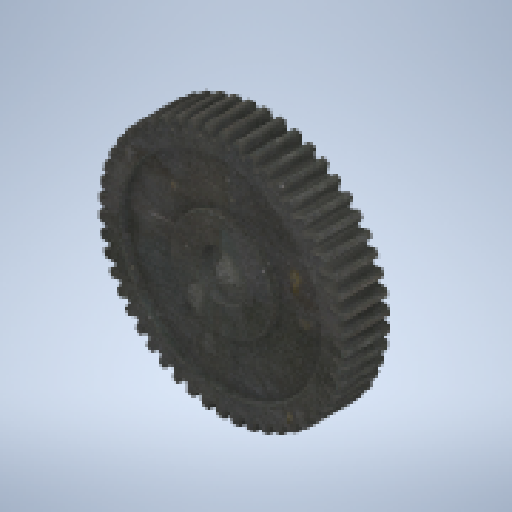
# Autodesk Inventor part: Engranaje recto2
Saved by Autodesk Inventor 2024 (Build 280153000, 153)
## iProperties
CustomPartVersion: 0
Created: 2023-12-10
Part Number: Engranaje recto2
Material: Acero
Document SubType Name: Modeling
Designer: Jhon
Categories: <?xml version="1.0" encoding="UTF-16"?> <MemberInstance><Categories><FamilyTemplate><FamilyTemplateParameter ValueType="xs:double" Id="1" ObjectReferenceKey="da_z" ObjectType="kUserParameterObject"/><FamilyTemplateParameter ValueType="xs:double" Id="2" ObjectReferenceKey="da_b" ObjectType="kUserParameterObject"/><FamilyTemplateParameter ValueType="xs:double" Id="3" ObjectReferenceKey="da_beta" ObjectType="kUserParameterObject"/><FamilyTemplateParameter ValueType="xs:double" Id="4" ObjectReferenceKey="da_da" ObjectType="kUserParameterObject"/><FamilyTemplateParameter ValueType="xs:double" Id="5" ObjectReferenceKey="da_aw" ObjectType="kUserParameterObject"/><FamilyTemplateParameter ValueType="xs:string" Id="6" ObjectReferenceKey="EAIAABAAAACIAQAAAAAAAIAAAAAAAAAA" ObjectType="83910656" SubObjectId="SurfaceGeometry"/></FamilyTemplate><ParamToTemplateMap><ParamToTemplate CategoryParameter="//CategoryParameter[@InternalName='046C89C9-8512-4d59-83FE-43B91F4F132A']" TemplateParameter="1"/><ParamToTemplate CategoryParameter="//CategoryParameter[@InternalName='2552DF32-E462-4b46-AEBF-C6C7768E72AC']" TemplateParameter="2"/><ParamToTemplate CategoryParameter="//CategoryParameter[@InternalName='C9EE641D-15FC-4fae-A226-E94C4372FDD7']" TemplateParameter="3"/><ParamToTemplate><ParamToTemplate CategoryParameter="//CategoryParameter[@InternalName='00B6519A-459B-49c7-AD84-2E56D39A5744']" ConstantValue="0.000000"/></ParamToTemplate><ParamToTemplate><ParamToTemplate CategoryParameter="//CategoryParameter[@InternalName='04B31F0E-C7A6-4894-AA32-9629BEFACF47']" ConstantValue="1.000000"/></ParamToTemplate><ParamToTemplate><ParamToTemplate CategoryParameter="//CategoryParameter[@InternalName='43CBEC2E-7847-49e7-A936-2F7889FCB2D9']" ConstantValue="0.250000"/></ParamToTemplate><ParamToTemplate><ParamToTemplate CategoryParameter="//CategoryParameter[@InternalName='B1EFC894-105D-4ebd-86BF-FA20ED196853']" ConstantValue="0.337200"/></ParamToTemplate><ParamToTemplate><ParamToTemplate CategoryParameter="//CategoryParameter[@InternalName='51175063-3D10-4879-93E8-6246FE8B403D']" ConstantValue="2060000000.000000"/></ParamToTemplate><ParamToTemplate><ParamToTemplate CategoryParameter="//CategoryParameter[@InternalName='A3A52E27-4454-46a9-B0BD-C932399B70AF']" ConstantValue="0.300000"/></ParamToTemplate><ParamToTemplate><ParamToTemplate CategoryParameter="//CategoryParameter[@InternalName='91B76062-C214-41d9-B1B9-14D2AB99603D']" ConstantValue="0.400000"/></ParamToTemplate><ParamToTemplate><ParamToTemplate CategoryParameter="//CategoryParameter[@InternalName='374E806E-8B8A-4dda-A9AA-1039D6500AD2']" ConstantValue="2.500000"/></ParamToTemplate><ParamToTemplate><ParamToTemplate CategoryParameter="//CategoryParameter[@InternalName='2D373A89-B862-43d6-8D0B-0CBF12AB9F6C']" ConstantValue="0.349066"/></ParamToTemplate><ParamToTemplate CategoryParameter="//CategoryParameter[@InternalName='37777632-D6A2-4fac-9D53-DB8ACD95C989']" TemplateParameter="4"/><ParamToTemplate CategoryParameter="//CategoryParameter[@InternalName='FD1017F1-B727-4f7e-9707-0F86F1FF9423']" TemplateParameter="5"/><ParamToTemplate><ParamToTemplate CategoryParameter="//CategoryParameter[@InternalName='9E1B4470-B2D3-4ff1-B813-535BB4CDF51A']" ConstantValue="3520000.000000"/></ParamToTemplate><ParamToTemplate><ParamToTemplate CategoryParameter="//CategoryParameter[@InternalName='F8452263-BFF6-458c-9FB1-07C4B99E95CD']" ConstantValue="11400000.000000"/></ParamToTemplate><ParamToTemplate><ParamToTemplate CategoryParameter="//CategoryParameter[@InternalName='3E3BB259-FD49-497f-8171-6EBC954A3479']" ConstantValue="2.000000"/></ParamToTemplate><ParamToTemplate CategoryParameter="//CategoryParameter[@InternalName='27C3BAF2-7550-4e4b-AE2C-0DB134B7D9B7']" TemplateParameter="6"/></ParamToTemplateMap><Category DisplayName="Gear" InternalName="DC85795E-93AB-48d5-8EEE-5A27447B64BD" Mnemonic="Gear"><CategoryParameter DisplayName="z" InternalName="046C89C9-8512-4d59-83FE-43B91F4F132A" Mnemonic="z"/><CategoryParameter DisplayName="b" InternalName="2552DF32-E462-4b46-AEBF-C6C7768E72AC" Mnemonic="b"/><CategoryParameter DisplayName="||b|" InternalName="C9EE641D-15FC-4fae-A226-E94C4372FDD7" Mnemonic="beta"/><CategoryParameter DisplayName="x" InternalName="00B6519A-459B-49c7-AD84-2E56D39A5744" Mnemonic="x"/><CategoryParameter DisplayName="a*" InternalName="04B31F0E-C7A6-4894-AA32-9629BEFACF47" Mnemonic="a"/><CategoryParameter DisplayName="c*" InternalName="43CBEC2E-7847-49e7-A936-2F7889FCB2D9" Mnemonic="c"/><CategoryParameter DisplayName="r|.f|*" InternalName="B1EFC894-105D-4ebd-86BF-FA20ED196853" Mnemonic="rf"/><CategoryParameter DisplayName="E" InternalName="51175063-3D10-4879-93E8-6246FE8B403D" Mnemonic="E"/><CategoryParameter DisplayName="||m|" InternalName="A3A52E27-4454-46a9-B0BD-C932399B70AF" Mnemonic="mi"/><Category DisplayName="SpurGear" InternalName="26C5A22E-A91E-4dfd-A3B3-23CCAFAE1764" Mnemonic="SpurGear"><CategoryParameter DisplayName="m" InternalName="91B76062-C214-41d9-B1B9-14D2AB99603D" Mnemonic="m"/><CategoryParameter DisplayName="P" InternalName="374E806E-8B8A-4dda-A9AA-1039D6500AD2" Mnemonic="PP"/><CategoryParameter DisplayName="||a|" InternalName="2D373A89-B862-43d6-8D0B-0CBF12AB9F6C" Mnemonic="alpha"/><CategoryParameter DisplayName="d|.a|" InternalName="37777632-D6A2-4fac-9D53-DB8ACD95C989" Mnemonic="da"/><CategoryParameter DisplayName="a|.w|" InternalName="FD1017F1-B727-4f7e-9707-0F86F1FF9423" Mnemonic="aw"/><CategoryParameter DisplayName="||s||.Flim|" InternalName="9E1B4470-B2D3-4ff1-B813-535BB4CDF51A" Mnemonic="sFlim"/><CategoryParameter DisplayName="||s||.Hlim|" InternalName="F8452263-BFF6-458c-9FB1-07C4B99E95CD" Mnemonic="sHlim"/><CategoryParameter DisplayName="tipo" InternalName="3E3BB259-FD49-497f-8171-6EBC954A3479" Mnemonic="type"/><CategoryParameter DisplayName="PitchDiameter" InternalName="27C3BAF2-7550-4e4b-AE2C-0DB134B7D9B7" Mnemonic="IDS_PITCHDIAM"/></Category></Category></Categories></MemberInstance>
Mass: 8265.26 g
Surface Area: 1323.38 cm^2
Volume: 1052.9 cm^3
Density: 7.85 g/cm^3
Appearance: Placa
Author: Jhon
Autodesk Inventor part; units mm, degrees
sketch "Sketch1" plane through (0, 0, 0) normal (0, 0, 1) x (1, 0, 0)
  circle A0 centre (0, 0) radius 104
  dimension "d0" = 208
  constraints: 1 centre point
  measures "d0" diameter of A0
extrude "Extrusion1" add sketch "Sketch1" along normal blind 40
ref_plane "Work Plane2" through (0, 0, 20) normal (0, 0, 1) x (1, 0, 0)
sketch "Sketch2" plane through (0, 0, 0) normal (0, 0, -1) x (-1, 0, 0)
  circle A0 centre (0, 0) radius 104 projected
  circle A1 centre (0, 0) radius 100
  dimension "d3" = 200
  constraints: 1 centre point, 1 coincident
  measures "d3" diameter of A1
surface extrude "Diámetro de separación" sketch "Sketch2" against normal through all shown no curves A1
ref_plane "Work Plane8" through (0, 0, 0) normal (0.9980267, 0.0627905, 0) x (0, 0, 1)
ref_plane "Work Plane9" through (0, 0, 0) normal (1, 0, 0) x (0, 1, 0)
spur gear teeth "Engranaje recto" teeth 50 pitch diameter 200 tip diameter 208 root diameter 190 face width 40 start plane through (0, 0, 0) normal (0, 0, -1) x (-1, 0, 0)
sketch "Boceto3" plane through (0, 0, 0) normal (0, 0, -1) x (-1, 0, 0)
  arc A0 (-18.0702, -8.5714) -> (-18.0702, 8.5714) centre (0, 0) ccw
  circle A1 centre (0, 0) radius 42.5
  circle A2 centre (0, 0) radius 84
  line L0 (-22.721, -8.5714) -> (-18.0702, -8.5714)
  line L1 (-18.0702, 8.5714) -> (-22.721, 8.5714)
  line L2 (-22.721, 8.5714) -> (-22.721, -8.5714)
  dimension "d49" = 40
  dimension "d50" = 85
  dimension "d53" = 168
  constraints: 6 end point, 3 centre point, 3 coincident, 2 point on circle, 1 horizontal, 1 parallel
  measures "d49" diameter of A0
  measures "d50" diameter of A1
  measures "d53" diameter of A2
sketch "Boceto5" plane through (0, 0, 40) normal (0, 0, 1) x (1, 0, 0)
  circle A0 centre (0, 0) radius 84
  circle A1 centre (0, 0) radius 42.5
  dimension "d67" = 168
  dimension "d68" = 85
  constraints: 2 centre point, 2 coincident
  measures "d67" diameter of A0
  measures "d68" diameter of A1
extrude "Extrusión6" add sketch "Boceto3" along normal blind 20 contours A1
extrude "Extrusión7" cut sketch "Boceto3" against normal blind 40 contours L0 L2 L1 A0
extrude "Extrusión8" cut sketch "Boceto3" against normal blind 7 contours A2
extrude "Extrusión9" cut sketch "Boceto5" against normal blind 7
chamfer "Chaflán2" distance 2 angle 45 50 edges at (103.7948, 6.5302, 0) (103.7948, -6.5302, 0) (102.1579, 19.4877, 0) (102.1579, -19.4877, 0) (98.9099, 32.1378, 0) (98.9099, -32.1378, 0) (94.102, 44.281, 0) (94.102, -44.281, 0) (87.8101, 55.726, 0) (87.8101, -55.726, 0) (80.1334, 66.2921, 0) (80.1334, -66.2921, 0) (71.1929, 75.8127, 0) (71.1929, -75.8127, 0) (61.1297, 84.1378, 0) (61.1297, -84.1378, 0) (50.1024, 91.1359, 0) (50.1024, -91.1359, 0) (38.285, 96.6968, 0) (38.285, -96.6968, 0) (25.8637, 100.7326, 0) (25.8637, -100.7326, 0) (13.0347, 103.1799, 0) (13.0347, -103.1799, 0) (0, 104, 0) (0, -104, 0) (-13.0347, 103.1799, 0) (-13.0347, -103.1799, 0) (-25.8637, 100.7326, 0) (-25.8637, -100.7326, 0) (-38.285, 96.6968, 0) (-38.285, -96.6968, 0) (-50.1024, 91.1359, 0) (-50.1024, -91.1359, 0) (-61.1297, 84.1378, 0) (-61.1297, -84.1378, 0) (-71.1929, 75.8127, 0) (-71.1929, -75.8127, 0) (-80.1334, 66.2921, 0) (-80.1334, -66.2921, 0) (-87.8101, 55.726, 0) (-87.8101, -55.726, 0) (-94.102, 44.281, 0) (-94.102, -44.281, 0) (-98.9099, 32.1378, 0) (-98.9099, -32.1378, 0) (-102.1579, 19.4877, 0) (-102.1579, -19.4877, 0) (-103.7948, 6.5302, 0) (-103.7948, -6.5302, 0)
chamfer "Chaflán3" distance 2 angle 45 50 edges at (103.7948, 6.5302, 40) (103.7948, -6.5302, 40) (102.1579, 19.4877, 40) (102.1579, -19.4877, 40) (98.9099, 32.1378, 40) (98.9099, -32.1378, 40) (94.102, 44.281, 40) (94.102, -44.281, 40) (87.8101, 55.726, 40) (87.8101, -55.726, 40) (80.1334, 66.2921, 40) (80.1334, -66.2921, 40) (71.1929, 75.8127, 40) (71.1929, -75.8127, 40) (61.1297, 84.1378, 40) (61.1297, -84.1378, 40) (50.1024, 91.1359, 40) (50.1024, -91.1359, 40) (38.285, 96.6968, 40) (38.285, -96.6968, 40) (25.8637, 100.7326, 40) (25.8637, -100.7326, 40) (13.0347, 103.1799, 40) (13.0347, -103.1799, 40) (0, 104, 40) (0, -104, 40) (-13.0347, 103.1799, 40) (-13.0347, -103.1799, 40) (-25.8637, 100.7326, 40) (-25.8637, -100.7326, 40) (-38.285, 96.6968, 40) (-38.285, -96.6968, 40) (-50.1024, 91.1359, 40) (-50.1024, -91.1359, 40) (-61.1297, 84.1378, 40) (-61.1297, -84.1378, 40) (-71.1929, 75.8127, 40) (-71.1929, -75.8127, 40) (-80.1334, 66.2921, 40) (-80.1334, -66.2921, 40) (-87.8101, 55.726, 40) (-87.8101, -55.726, 40) (-94.102, 44.281, 40) (-94.102, -44.281, 40) (-98.9099, 32.1378, 40) (-98.9099, -32.1378, 40) (-102.1579, 19.4877, 40) (-102.1579, -19.4877, 40) (-103.7948, 6.5302, 40) (-103.7948, -6.5302, 40)
chamfer "Chaflán4" distance 1 angle 45 10 edges at (84, 0, 0) (84, 0, 7) (42.5, 0, -20) (42.5, 0, 7) (-20, 0, -20) (-84, 0, 40) (-84, 0, 33) (-42.5, 0, 40) (-42.5, 0, 33) (-20, 0, 40)
equation "\"d0\" = da_da"
equation "\"d1\" = da_b"
equation "\"d3\" = da_d"
equation "\"da_da\" = 208"
equation "\"da_b\" = 40"
equation "\"da_d\" = 200"
body "Solid1"
body "Srf1"
